lack_table_join (Autodesk Fusion 360 design; units mm, degrees)
Autodesk Fusion 360 part; units mm, degrees
sketch "Sketch1" plane through (0, 0, 0) normal (0, 0, 1) x (1, 0, 0)
  line L0 (0, 0) -> (-50.6, 0)
  line L1 (-50.6, 0) -> (-50.6, 50.6)
  line L2 (-50.6, 50.6) -> (0, 50.6)
  line L3 (0, 50.6) -> (0, 0)
  line L4 (3, -3) -> (-53.6, -3)
  line L5 (-53.6, -3) -> (-53.6, 53.6)
  line L6 (-53.6, 53.6) -> (3, 53.6)
  line L7 (3, 53.6) -> (3, -3)
  line L8 (-50.6, 0) -> (-52.4, 0)
  line L9 (-52.4, 0) -> (-52.4, 52.4)
  line L10 (-52.4, 52.4) -> (0, 52.4)
  line L11 (0, 52.4) -> (0, 50.6)
  line L12 (0, 50.6) -> (3, 50.6)
  line L13 (3, 50.6) -> (3, 52.4)
  line L14 (3, 52.4) -> (0, 52.4)
  line L15 (0, 52.4) -> (0, 50.6)
  line L16 (-50.6, 0) -> (-52.4, 0)
  line L17 (-52.4, 0) -> (-52.4, -3)
  line L18 (-52.4, -3) -> (-50.6, -3)
  line L19 (-50.6, -3) -> (-50.6, 0)
  line L20 (3, 55.4) -> (0, 55.4)
  line L21 (-55.4, 55.4) -> (0, 55.4)
  line L22 (-55.4, 0) -> (-55.4, 55.4)
  line L23 (-55.4, 0) -> (-55.4, -3)
  line L24 (3, 55.4) -> (3, 53.6)
  line L25 (-55.4, -3) -> (-53.6, -3)
  dimension "d1" = 50.6
  dimension "d2" = 50.6
  dimension "d3" = -3
  dimension "d6" = 1.8
  dimension "d7" = 1.8
  dimension "d8" = 3
  constraint horizontal L0
  constraint vertical L1
  constraint horizontal L2
  constraint vertical L3
  constraint coincident L0.start L3.end
  constraint perpendicular L1 L8
  constraint perpendicular L8 L9
  constraint perpendicular L9 L10
  constraint collinear L3 L11
  constraint horizontal L12
  constraint vertical L13
  constraint horizontal L14
  constraint vertical L15
  constraint collinear L10 L14
  constraint collinear L7 L13
  constraint horizontal L16
  constraint vertical L17
  constraint horizontal L18
  constraint vertical L19
  constraint collinear L9 L17
  constraint collinear L4 L18
  constraint perpendicular L6 L24
  constraint perpendicular L5 L25
  measures "d1" distance of L0.start L2.end
  measures "d2" distance of L0.start L0.end
  measures "d6" distance of L1 L9
  measures "d7" distance of L2 L10
  measures "d8" distance of L14
extrude "Extrude1" add sketch "Sketch1" along normal blind 135 contours L0 L3 L4 L7 L12 L19 | L1 L2 L8 L9 L10 L11 L15 L16 | L4 L8 L16 L17 L18 L19 | L7 L11 L12 L13 L14 L15 | L4 L5 L6 L7 L9 L10 L14 L17 makes body 1
extrude "Extrude2" add sketch "Sketch1" along normal blind -40 and the other way blind -135 contours L4 L5 L6 L7 L9 L10 L14 L17 | L5 L6 L20 L21 L22 L23 L24 L25 bodies 1
extrude "Extrude3" add sketch "Sketch1" along normal blind 175 contours L0 L1 L2 L3 bodies 1
extrude "Extrude4" add 1 faces at (-53.8, 34.3333, 135) along direction (0, 0, 1) blind 60 on bodies 1 bodies 1
extrude "Extrude5" add 1 faces at (-16.8667, 16.8667, 175) along direction (0, 0, 1) blind 25 separate body on bodies 1 makes body 2
extrude "Extrude6" add 1 faces at (-53.8, 34.3333, 195) along direction (0, 0, 1) blind 25 separate body on bodies 1 makes body 3
combine "Combine1" operation add target body 2 tool bodies 3
move_face "OffsetFaces1" offset -0.2 4 faces at (-16.8667, 0, 181.6667) (0, 33.7333, 181.6667) (-33.7333, 50.6, 181.6667) (-50.6, 16.8667, 181.6667) on bodies 2
hidden bodies 1
equation "d2 = d1"
equation "d7 = d6"
